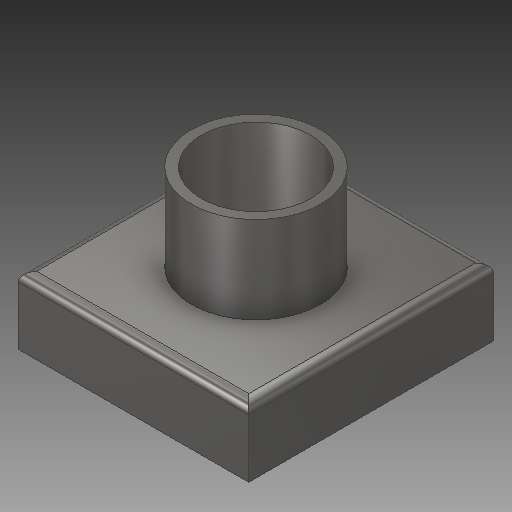
# Autodesk Inventor part: PEC12R-4017F-N0024 Base
Saved by Autodesk Inventor 2018 (Build 220112000, 112)
## iProperties
Created: 2018-01-11
Part Number: PEC12R-4017F-N0024 Base
Material: Generic
Document SubType Name: Modeling
Designer: Moochster
Density: 1 g/cm^3
Appearance: Semi-Polished
Mass: 0.674139 g
Surface Area: 7.13817 cm^2
Volume: 0.674139 cm^3
Author: Moochster
Autodesk Inventor part; units mm, degrees
ref_plane "YZ Plane" through (0, 0, 0) normal (1, 0, 0) x (0, 1, 0)
ref_plane "XZ Plane" through (0, 0, 0) normal (0, 1, 0) x (-1, 0, 0)
ref_plane "XY Plane" through (0, 0, 0) normal (0, 0, 1) x (1, 0, 0)
sketch "Sketch1" plane through (0, 0, 0) normal (0, 1, 0) x (-1, 0, 0)
  line L0 (0, 0) -> (-12.6, 0)
  line L1 (-12.6, 0) -> (-12.6, -13.4)
  line L2 (-12.6, -13.4) -> (0, -13.4)
  line L3 (0, -13.4) -> (0, 0)
  dimension "d0" = 12.6
  dimension "d1" = 13.4
  constraints: 8 end point, 2 parallel, 1 horizontal, 1 perpendicular
  measures "d0" distance of L2.end L1.end
  measures "d1" distance of L1.end L0.end
extrude "Extrusion1" add sketch "Sketch1" along normal blind 3.7
sketch "Sketch2" plane through (0, 3.7, 0) normal (0, 1, 0) x (1, 0, 0)
  circle A0 centre (6.3, 6.7) radius 3.535
  line L0 (12.6, 13.4) -> (0, 13.4) projected
  line L1 (12.6, 0) -> (12.6, 13.4) projected
  circle A1 centre (6.3, 6.7) radius 3
  point P0 (0, 0)
  point P1 (6.3, 13.4)
  point P2 (12.6, 6.7)
  dimension "d4" = 7.07
  dimension "d17" = 6
  constraints: 2 centre point, 2 midpoint, 1 coincident, 1 horizontal alignment, 1 vertical alignment
  measures "d4" diameter of A0
  measures "d17" diameter of A1
extrude "Extrusion2" add sketch "Sketch2" along normal blind 4.75
fillet "Fillet1" radius 0.5 4 edges at (6.3, 3.7, 0) (12.6, 3.7, -6.7) (6.3, 3.7, -13.4) (0, 3.7, -6.7)
sketch "Sketch3" plane through (6.3, 8.45, -6.7) normal (0, 1, 0) x (1, 0, 0)
  circle A0 centre (0, 0) radius 3
  circle A1 centre (0, 0) radius 3.535 projected
  point P0 (-6.3, -6.7)
  dimension "d7" = 6
  constraints: 1 centre point, 1 concentric
  measures "d7" diameter of A0
sketch "Sketch4" plane through (6.3, 15.9, -6.7) normal (0, 1, 0) x (1, 0, 0)
  line L0 (1.46, 3.1507) -> (1.46, -2.6208)
  circle A0 centre (0, 0) radius 3 construction
  point P0 (-6.3, -6.7)
  point P1 (-3, 0)
  dimension "d13" = 4.46
  constraints: 2 end point, 2 point on circle, 1 horizontal alignment, 1 vertical
  measures "d13" distance from line of L0 A0.end
body "Solid1"
